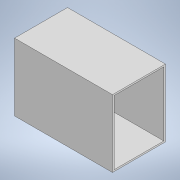
# Autodesk Inventor part: battery and buck converter enclosure
Saved by Autodesk Inventor 2022 (Build 260153000, 153)
## iProperties
Created: 2021-10-07
Part Number: battery and buck converter enclosure
Material: Generic
Document SubType Name: Modeling
Designer: tecware
Density: 1 g/cm^3
Appearance: Default
Author: tecware
Autodesk Inventor part; units mm, degrees
ref_plane "YZ Plane" through (0, 0, 0) normal (1, 0, 0) x (0, 1, 0)
ref_plane "XZ Plane" through (0, 0, 0) normal (0, 1, 0) x (-1, 0, 0)
ref_plane "XY Plane" through (0, 0, 0) normal (0, 0, 1) x (1, 0, 0)
sketch "Sketch1" plane through (0, 0, 0) normal (0, 1, 0) x (-1, 0, 0)
  line L0 (30, -15.5) -> (-30, -15.5)
  line L1 (-30, -15.5) -> (-30, 15.5)
  line L2 (-30, 15.5) -> (30, 15.5)
  line L3 (30, 15.5) -> (30, -15.5)
  dimension "d0" = 60
  dimension "d1" = 31
  constraints: 8 end point, 2 parallel, 1 horizontal, 1 perpendicular
  measures "d0" distance of L1.end L2.end
  measures "d1" distance of L0.end L1.end
extrude "Extrusion1" add sketch "Sketch1" along normal blind 40
shell "Shell1" thickness 1 outward yes removed faces 1 at (30, 13.3333, 5.1667)
body "Solid1"
